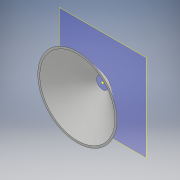
# Autodesk Inventor part: DPLX_P010_Wire_Mesh_reducer_Spark_Gap
Saved by Autodesk Inventor 2018 (Build 220112000, 112)
## iProperties
Created: 2018-06-07
Part Number: DPLX_P010_Wire_Mesh_reducer_Spark_Gap
Material: Generic
Document SubType Name: Modeling
Designer: DPLXuser
Density: 1 g/cm^3
Appearance: Default
Author: DPLXuser
Autodesk Inventor part; units mm, degrees
ref_plane "YZ Plane" through (0, 0, 0) normal (1, 0, 0) x (0, 1, 0)
ref_plane "XY Plane" through (0, 0, 0) normal (0, 0, 1) x (1, 0, 0)
sketch "Sketch1" plane through (0, 0, 0) normal (0, 1, 0) x (-1, 0, 0)
  circle A0 centre (0, 0) radius 15.7085
  dimension "d0" = 31.417
  constraints: 1 centre point, 1 coincident
  measures "d0" diameter of A0
ref_plane "Work Plane1" through (0, 10, 0) normal (0, 1, 0) x (-1, 0, 0)
sketch "Sketch3" plane through (0, 10, 0) normal (0, 1, 0) x (-1, 0, 0)
  point P0 (0, 0)
sketch "Sketch4" plane through (0, 10, 0) normal (0, 1, 0) x (-1, 0, 0)
  circle A0 centre (0, 0) radius 3.175
  dimension "d8" = 6.35
  constraints: 1 centre point, 1 coincident
  measures "d8" diameter of A0
loft "Loft2" add profiles "Sketch1", "Sketch4"
shell "Shell2" thickness 0.5 removed faces 2 at (0.5202, 10, -0.7796) at (2.3044, 0, 8.5824)
body "Solid2"
